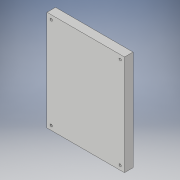
# Autodesk Inventor part: arduinoCover
Saved by Autodesk Inventor 2017 (Build 210142000, 142)
## iProperties
Created: 2017-04-16
Part Number: arduinoCover
Material: Generic
Document SubType Name: Modeling
Designer: rocke
Density: 1 g/cm^3
Appearance: Default
Author: rocke
Autodesk Inventor part; units mm, degrees
ref_plane "YZ Plane" through (0, 0, 0) normal (1, 0, 0) x (0, 1, 0)
ref_plane "XZ Plane" through (0, 0, 0) normal (0, 1, 0) x (-1, 0, 0)
ref_plane "XY Plane" through (0, 0, 0) normal (0, 0, 1) x (1, 0, 0)
sketch "Sketch1" plane through (0, 0, 0) normal (0, 0, 1) x (1, 0, 0)
  line L0 (0, 0) -> (68.834, 0)
  line L1 (68.834, 0) -> (68.834, 89.027)
  line L2 (68.834, 89.027) -> (0, 89.027)
  line L3 (0, 89.027) -> (0, 0)
  dimension "d0" = 89.027
  dimension "d1" = 68.834
  constraints: 8 end point, 2 parallel, 1 horizontal, 1 perpendicular
  measures "d0" distance of L0.end L1.end
  measures "d1" distance of L1.end L2.end
extrude "Extrusion1" add sketch "Sketch1" along normal blind 7.62
sketch "Sketch2" plane through (0, 0, 7.62) normal (0, 0, 1) x (1, 0, 0)
  line L0 (68.834, 89.027) -> (0, 89.027) projected
  line L1 (0, 89.027) -> (3.81, 89.027)
  line L2 (3.81, 89.027) -> (3.81, 85.216)
  line L3 (3.81, 85.216) -> (0, 85.216)
  line L4 (0, 85.216) -> (0, 89.027)
  circle A0 centre (3.81, 85.216) radius 1.0414
  line L5 (68.834, 89.027) -> (65.024, 89.027)
  line L6 (65.024, 89.027) -> (65.024, 85.216)
  line L7 (65.024, 85.216) -> (68.834, 85.216)
  line L8 (68.834, 85.216) -> (68.834, 89.027)
  circle A1 centre (65.024, 85.216) radius 1.0414
  line L9 (0, 0) -> (68.834, 0) projected
  line L10 (68.834, 0) -> (65.024, 0)
  line L11 (65.024, 0) -> (65.024, 3.8136)
  line L12 (65.024, 3.8136) -> (68.834, 3.8136)
  line L13 (68.834, 3.8136) -> (68.834, 0)
  circle A2 centre (65.024, 3.8136) radius 1.0414
  line L14 (0, 0) -> (3.81, 0)
  line L15 (3.81, 0) -> (3.81, 3.8136)
  line L16 (3.81, 3.8136) -> (0, 3.8136)
  line L17 (0, 3.8136) -> (0, 0)
  circle A3 centre (3.81, 3.8136) radius 1.0414
  dimension "d4" = 3.81
  dimension "d5" = 2.0828
  dimension "d6" = 3.81
  dimension "d7" = 2.0828
  dimension "d8" = 2.0828
  dimension "d9" = 2.0828
  constraints: 32 end point, 8 parallel, 4 centre point, 4 coincident, 4 horizontal, 4 perpendicular
  measures "d4" distance of L2.end L3.end
  measures "d5" diameter of A0
  measures "d6" distance of L7.end L6.end
  measures "d7" diameter of A1
  measures "d8" diameter of A2
  measures "d9" diameter of A3
extrude "Extrusion2" cut sketch "Sketch2" against normal blind 7.62 contours A0 L3 L2 | L2 L3 A0
extrude "Extrusion3" cut sketch "Sketch2" against normal blind 7.62 contours A1 L7 L6 | L6 L7 A1
extrude "Extrusion4" cut sketch "Sketch2" against normal blind 7.62 contours A2 L12 L11 | L11 L12 A2
extrude "Extrusion5" cut sketch "Sketch2" against normal blind 7.62 contours A3 L16 L15 | L15 L16 A3
body "Solid1"
